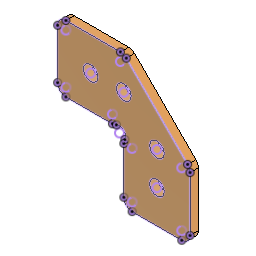
Custom Short L-Bracket (Autodesk Fusion 360 design; units mm, degrees)
Autodesk Fusion 360 part; units mm, degrees
sketch "Sketch1" plane through (0, 0, 0) normal (0, 1, 0) x (1, 0, 0)
  line L0 (0, 0) -> (0, -25.4)
  line L1 (76.2, -25.4) -> (76.2, 0)
  line L2 (76.2, 0) -> (50.8, 0)
  line L3 (50.8, 0) -> (50.8, -25.4)
  line L4 (50.8, -25.4) -> (25.4, -25.4)
  line L5 (25.4, -25.4) -> (25.4, 0)
  line L6 (25.4, 0) -> (0, 0)
  line L7 (38.1, -25.4) -> (38.1, -50.8) construction
  circle A0 centre (27.0838, -23.7162) radius 2.3813
  line L8 (27.0838, -23.7162) -> (27.0838, -25.4) construction
  line L9 (27.0838, -23.7162) -> (25.4, -23.7162) construction
  circle A1 centre (12.7, -12.7) radius 2.7781
  line L10 (0, -25.4) -> (25.4, -50.8)
  line L11 (25.4, -50.8) -> (50.8, -50.8)
  line L12 (50.8, -50.8) -> (76.2, -25.4)
  circle A2 centre (12.7, -25.4) radius 2.7781
  circle A3 centre (25.4, -38.1) radius 2.7781
  circle A4 centre (38.1, -38.1) radius 2.7781
  circle A5 centre (50.8, -38.1) radius 2.7781
  circle A6 centre (63.5, -12.7) radius 2.7781
  circle A7 centre (63.5, -25.4) radius 2.7781
  circle A8 centre (49.1162, -23.7162) radius 2.3813
  dimension "d1" = 76.2
  dimension "d3" = 25.4
  dimension "d4" = 25.4
  dimension "d6" = 25.4
  dimension "d8" = 4.7625
  dimension "d9" = 5.5563
  dimension "d10" = 12.7
  dimension "d26" = 25.4
  dimension "d43" = 25.4
  dimension "d44" = 12.7
  dimension "d47" = -25.4
  dimension "d48" = -50.8
  constraint coincident L0.start L6.end
  constraint vertical L0
  constraint perpendicular L1 L2
  constraint perpendicular L2 L3
  constraint perpendicular L3 L4
  constraint perpendicular L4 L5
  constraint perpendicular L0 L6
  constraint equal L2 L6
  constraint midpoint L4 L7.start
  constraint equal L0 L1
  constraint coincident L4.end A0
  constraint coincident A0.centre L8.start
  constraint coincident L4 L8.end
  constraint perpendicular L4 L8
  constraint coincident L5 L9.end
  constraint perpendicular L5 L9
  constraint equal L8 L9
  constraint perpendicular L0 L11
  constraint equal L10 L12
  constraint collinear L2 L6
  constraint coincident L7.end L11
  constraint symmetric L7 A0 A8
  constraint midpoint L7.end L11
  measures "d1" distance of L0 L1
  measures "d3" distance of L3.end L4.end
  measures "d4" distance of L4.end L5.end
  measures "d6" distance of L0.start L0.end
  measures "d8" diameter of A0
  measures "d9" diameter of A1
  measures "d10" distance of L6 A1.centre
  measures "d26" distance of L10.end L11.end
  measures "d43" distance of L4 L11
  measures "d44" distance of L0 A1.centre
extrude "Extrude1" add sketch "Sketch1" along normal blind 3.175 contours L0 L1 L2 L3 L4 L5 L6 A0 L10 L11 L12 A8 | L5 A0 | L4 A0 | A1 | A2 | A3 makes body 1
ref_plane "WorkPlane1" through (25.4, 1.5875, 12.7) normal (-1, 0, 0) x (0, 0, 1)
split "Split1" by plane through (25.4, 1.5875, 12.7) normal (-1, 0, 0) bodies 1 makes body 2 at (8.4667, 0, 15.8108)
delete_body "RemoveBody1" bodies 2
fillet "Fillet1" radius 3.175 6 edges at (50.8, 1.5875, 0) (76.2, 1.5875, 0) (50.8, 1.5875, 50.8) (76.2, 1.5875, 25.4) (25.4, 1.5875, 25.4) (25.4, 1.5875, 50.8) on bodies 1
fillet "Fillet1" radius 3.175 2 edges at (47.4324, 1.5875, 25.4) (50.8, 1.5875, 22.0324) on bodies 1
sketch "DXF" plane through (0, 0, 0) normal (0, -1, 0) x (1, 0, 0)
  arc A0 (51.1985, 22.5611) -> (50.8, 21.021) centre (53.975, 21.021) ccw
  line L0 (50.8, 21.021) -> (50.8, 3.175)
  arc A1 (50.8, 3.175) -> (53.975, 0) centre (53.975, 3.175) ccw
  line L1 (53.975, 0) -> (73.025, 0)
  arc A2 (73.025, 0) -> (76.2, 3.175) centre (73.025, 3.175) ccw
  line L2 (76.2, 3.175) -> (76.2, 24.0849)
  arc A3 (76.2, 24.0849) -> (75.2701, 26.3299) centre (73.025, 24.0849) ccw
  line L3 (75.2701, 26.3299) -> (51.7299, 49.8701)
  arc A4 (51.7299, 49.8701) -> (49.4849, 50.8) centre (49.4849, 47.625) ccw
  line L4 (49.4849, 50.8) -> (28.575, 50.8)
  arc A5 (28.575, 50.8) -> (25.4, 47.625) centre (28.575, 47.625) ccw
  line L5 (25.4, 47.625) -> (25.4, 28.575)
  arc A6 (25.4, 28.575) -> (28.575, 25.4) centre (28.575, 28.575) ccw
  line L6 (28.575, 25.4) -> (46.421, 25.4)
  arc A7 (46.421, 25.4) -> (47.9611, 25.7985) centre (46.421, 28.575) ccw
  arc A8 (51.1985, 22.5611) -> (47.9611, 25.7985) centre (49.1162, 23.7162) ccw
  circle A9 centre (38.1, 38.1) radius 2.7781
  circle A10 centre (50.8, 38.1) radius 2.7781
  circle A11 centre (63.5, 12.7) radius 2.7781
  circle A12 centre (63.5, 25.4) radius 2.7781
equation "TOLERANCE = 0 in" comment "Tube size tolerance"
equation "d3 = 1 in + TOLERANCE"
equation "d9 = ( 7 / 32 ) * 1 in"
